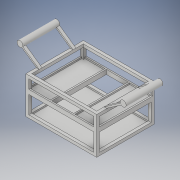
# Autodesk Inventor part: Battery Cart
Saved by Autodesk Inventor 2019.4 (Build 234330000, 330)
## iProperties
Created: 2019-09-11
Part Number: Battery Cart
Material: Generic
Document SubType Name: Modeling
Designer: josh
Density: 1 g/cm^3
Appearance: Default
Author: josh
Autodesk Inventor part; units mm, degrees
sketch "Sketch1" plane through (0, 0, 0) normal (1, 0, 0) x (0, 1, 0)
  line L0 (0, 0) -> (141.732, 0)
  line L1 (141.732, 0) -> (141.732, -495.3)
  line L2 (141.732, -495.3) -> (0, -495.3)
  line L3 (0, -495.3) -> (0, 0)
  dimension "d0" = 495.3
  dimension "d1" = 141.732
  constraints: 8 end point, 2 parallel, 1 horizontal, 1 perpendicular
  measures "d0" distance of L0.end L1.end
  measures "d1" distance of L1.end L2.end
extrude "Extrusion1" add sketch "Sketch1" along normal blind 609.6
shell "Shell1" thickness 25.4 removed faces 1 at (203.2, 141.732, -165.1)
sketch "Sketch2" plane through (0, 0, 0) normal (0, 0, 1) x (1, 0, 0)
  line L0 (25.4, 25.4) -> (25.4, 141.732) projected
  line L1 (584.2, 141.732) -> (584.2, 25.4) projected
  line L2 (25.4, 25.4) -> (584.2, 25.4)
  line L3 (584.2, 25.4) -> (584.2, 116.332)
  line L4 (584.2, 116.332) -> (25.4, 116.332)
  line L5 (25.4, 116.332) -> (25.4, 25.4)
  point P0 (0, 0)
  dimension "d5" = 90.932
  constraints: 8 end point, 2 parallel, 1 horizontal, 1 perpendicular, 1 point on line
  measures "d5" distance of L3.end L2.end
sketch "Sketch4" plane through (0, 0, 0) normal (-1, 0, 0) x (0, 0, 1)
  line L0 (-25.4, 141.732) -> (-25.4, 25.4) projected
  line L1 (-469.9, 25.4) -> (-469.9, 141.732) projected
  line L2 (-25.4, 25.4) -> (-469.9, 25.4)
  line L3 (-469.9, 25.4) -> (-469.9, 116.332)
  line L4 (-469.9, 116.332) -> (-25.4, 116.332)
  line L5 (-25.4, 116.332) -> (-25.4, 25.4)
  point P0 (0, 0)
  dimension "d13" = 90.932
  constraints: 8 end point, 2 parallel, 1 horizontal, 1 perpendicular, 1 point on line
  measures "d13" distance of L2.end L3.end
extrude "Extrusion6" cut sketch "Sketch4" against normal through all
extrude "Extrusion7" cut sketch "Sketch2" against normal through all
sketch "Sketch9" plane through (609.6, 25.4, -25.4) normal (0, 1, 0) x (1, 0, 0)
  line L0 (-609.6, -25.4) -> (-609.6, 469.9) projected
  line L1 (-609.6, 469.9) -> (0, 469.9) projected
  line L2 (0, 469.9) -> (0, -25.4) projected
  line L3 (-609.6, -25.4) -> (0, -25.4) projected
  line L4 (-609.6, 444.5) -> (-584.2, 444.5) projected
  line L5 (-596.9, 444.5) -> (-596.9, 0)
  line L6 (-609.6, 0) -> (-584.2, 0) projected
  line L7 (-584.2, 444.5) -> (-584.2, 469.9) projected
  line L8 (-584.2, 457.2) -> (-25.4, 457.2)
  line L9 (-25.4, 444.5) -> (-25.4, 469.9) projected
  line L10 (-25.4, 444.5) -> (0, 444.5) projected
  line L11 (-12.7, 444.5) -> (-12.7, 0)
  line L12 (-25.4, 0) -> (0, 0) projected
  line L13 (-584.2, -25.4) -> (-584.2, 0) projected
  line L14 (-584.2, -12.7) -> (-25.4, -12.7)
  line L15 (-25.4, -25.4) -> (-25.4, 0) projected
  line L16 (-609.6, 444.5) -> (-584.2, 444.5) projected
  line L17 (-596.9, 444.5) -> (-609.6, 444.5)
  line L18 (-609.6, 0) -> (-596.9, 0)
  line L19 (-609.6, 0) -> (-584.2, 0) projected
  line L20 (-25.4, 457.2) -> (-25.4, 469.9)
  line L21 (-609.6, 469.9) -> (0, 469.9) projected
  line L22 (-25.4, 444.5) -> (0, 444.5) projected
  line L23 (-12.7, 444.5) -> (0, 444.5)
  line L24 (-25.4, 457.2) -> (-25.4, 469.9)
  line L25 (-25.4, 0) -> (0, 0) projected
  line L26 (-12.7, 0) -> (0, 0)
  line L27 (-25.4, -12.7) -> (-25.4, -25.4)
  line L28 (-25.4, -25.4) -> (-584.2, -25.4) projected
  line L29 (-584.2, -25.4) -> (-584.2, -12.7)
  line L30 (-609.6, 444.5) -> (-609.6, 0)
  line L31 (-609.6, 469.9) -> (-609.6, -25.4) projected
  line L32 (-584.2, -25.4) -> (-25.4, -25.4)
  line L33 (-584.2, 469.9) -> (-25.4, 469.9) projected
  line L34 (-25.4, 469.9) -> (-584.2, 469.9)
  line L35 (0, 444.5) -> (0, 0) projected
  line L36 (0, 444.5) -> (0, 0)
  constraints: 32 end point, 8 midpoint, 6 collinear, 3 perpendicular, 2 horizontal, 1 parallel
extrude "Extrusion14" add sketch "Sketch9" along normal blind 12.7 contours L0 L4 L5 L6 | L13 L14 L15 L3 | L0 L1 L7 L4 | L1 L9 L8 L7 | L12 L11 L10 L2 | L1 L2 L10 L9
sketch "Sketch10" plane through (0, 0, -495.3) normal (0, -1, 0) x (1, 0, 0)
  line L0 (25.4, 469.9) -> (25.4, 25.4) projected
  line L1 (0, 495.3) -> (25.4, 495.3)
  line L2 (25.4, 495.3) -> (25.4, 469.9)
  line L3 (25.4, 469.9) -> (0, 469.9)
  line L4 (0, 469.9) -> (0, 495.3)
  line L5 (25.4, 25.4) -> (0, 25.4)
  line L6 (0, 25.4) -> (0, 0)
  line L7 (0, 0) -> (25.4, 0)
  line L8 (25.4, 0) -> (25.4, 25.4)
  line L9 (609.6, 0) -> (609.6, 495.3) projected
  line L10 (609.6, 0) -> (584.2, 0)
  line L11 (584.2, 0) -> (584.2, 25.4)
  line L12 (584.2, 25.4) -> (609.6, 25.4)
  line L13 (609.6, 25.4) -> (609.6, 0)
  line L14 (584.2, 469.9) -> (25.4, 469.9) projected
  line L15 (609.6, 495.3) -> (584.2, 495.3)
  line L16 (584.2, 495.3) -> (584.2, 469.9)
  line L17 (584.2, 469.9) -> (609.6, 469.9)
  line L18 (609.6, 469.9) -> (609.6, 495.3)
  dimension "d48" = 25.4
  dimension "d49" = 25.4
  dimension "d50" = 25.4
  dimension "d51" = 25.4
  dimension "d52" = 25.4
  dimension "d53" = 25.4
  dimension "d54" = 25.4
  dimension "d55" = 25.4
  constraints: 32 end point, 8 parallel, 4 horizontal, 4 perpendicular
  measures "d48" distance of L0.start L3.end
  measures "d49" distance of L1.end L0.start
  measures "d50" distance of L7.end L6.end
  measures "d51" distance of L6.end L5.end
  measures "d52" distance of L11.end L12.end
  measures "d53" distance of L10.end L11.end
  measures "d54" distance of L17.end L14.start
  measures "d55" distance of L14.start L15.end
extrude "Extrusion15" add sketch "Sketch10" along normal blind 152.4
sketch "Sketch11" plane through (0, -152.4, -495.3) normal (0, -1, 0) x (1, 0, 0)
  line L0 (609.6, 0) -> (609.6, 25.4) projected
  line L1 (0, 495.3) -> (609.6, 495.3)
  line L2 (609.6, 495.3) -> (609.6, 0)
  line L3 (609.6, 0) -> (0, 0)
  line L4 (0, 0) -> (0, 495.3)
  constraints: 8 end point, 2 parallel, 1 horizontal, 1 perpendicular
extrude "Extrusion16" add sketch "Sketch11" along normal blind 25.4
sketch "Sketch12" plane through (25.4, 25.4, -12.7) normal (0, 1, 0) x (1, 0, 0)
  line L0 (185.42, 457.2) -> (185.42, 12.7)
  line L1 (373.38, 457.2) -> (373.38, 12.7)
  line L2 (373.38, 457.2) -> (373.38, 12.7)
  line L3 (185.42, 12.7) -> (185.42, 457.2)
  line L4 (373.38, 457.2) -> (373.38, 469.9)
  line L5 (185.42, 469.9) -> (185.42, 457.2)
  line L6 (185.42, 12.7) -> (185.42, 1.0295)
  line L7 (373.38, 1.0295) -> (373.38, 12.7)
  line L8 (185.42, 469.9) -> (373.38, 469.9)
  line L9 (373.38, 469.9) -> (373.38, 1.0295)
  line L10 (373.38, 1.0295) -> (185.42, 1.0295)
  line L11 (185.42, 1.0295) -> (185.42, 469.9)
  line L12 (558.8, 0) -> (0, 0) projected
  line L13 (185.42, 469.9) -> (172.72, 469.9)
  line L14 (172.72, 469.9) -> (172.72, 0)
  line L15 (172.72, 0) -> (185.42, 0)
  line L16 (185.42, 0) -> (185.42, 469.9)
  line L17 (373.38, 469.9) -> (386.08, 469.9)
  line L18 (386.08, 469.9) -> (386.08, -5.7755)
  line L19 (386.08, -5.7755) -> (373.38, -5.7755)
  line L20 (373.38, -5.7755) -> (373.38, 469.9)
  dimension "d64" = 12.7
  dimension "d65" = 12.7
  constraints: 40 end point, 9 parallel, 3 horizontal, 3 perpendicular, 2 point on line
  measures "d64" distance of L15.end L14.end
  measures "d65" distance of L18.end L19.end
extrude "Extrusion17" cut sketch "Sketch12" against normal blind 25.4 contours L5 L8 L4 L1 L7 L10 L6 L0
extrude "Extrusion18" add sketch "Sketch12" along normal blind 12.7 contours L0 L6 L16 L12 L14 L13 L5 | L17 L18 L12 L20 L7 L1 L4 | L12 L18 L19 L20
sketch "Sketch13" plane through (0, -152.4, -495.3) normal (0, 1, 0) x (1, 0, 0)
  line L0 (609.6, -495.3) -> (0, -495.3) projected
  line L1 (609.6, 0) -> (609.6, -495.3) projected
  line L2 (0, -495.3) -> (0, 0) projected
  line L3 (0, 0) -> (609.6, 0) projected
  line L4 (584.2, -25.4) -> (584.2, -469.9)
  line L5 (584.2, -469.9) -> (25.4, -469.9)
  line L6 (25.4, -469.9) -> (25.4, -25.4)
  line L7 (25.4, -25.4) -> (584.2, -25.4)
  dimension "d68" = 25.4
  constraints: 8 end point, 3 other
  measures "d68" distance between parallel lines of L3 L7
extrude "Extrusion19" cut sketch "Sketch13" against normal blind 12.7 contours L4 L5 L6 L7
ref_plane "Work Plane1" through (609.6, 141.732, -393.7) normal (0, 0, -1) x (-1, 0, 0)
ref_plane "Work Plane2" through (0, 141.732, -101.6) normal (0, 0, 1) x (1, 0, 0)
sketch "Sketch14" plane through (0, 141.732, -101.6) normal (0, 0, 1) x (1, 0, 0)
  line L0 (584.2, 0) -> (25.4, 0) projected
  line L1 (16.946, -12.0735) -> (25.4, 0)
  line L2 (25.4, 0) -> (228.6, 0) construction
  line L3 (25.4, 0) -> (-141.0517, 116.5507)
  line L4 (-141.0517, 116.5507) -> (-148.3361, 106.1475)
  line L5 (-148.3361, 106.1475) -> (18.1156, -10.4032)
  line L6 (18.1156, -10.4032) -> (25.4, 0)
  line L7 (25.4, 0) -> (228.6, 0) construction
  point P0 (0, -141.732)
  dimension "d75" = 203.2
  dimension "d76" = 145
  dimension "d77" = 12.7
  constraints: 14 end point, 2 horizontal, 2 parallel, 1 equal length, 1 perpendicular
  measures "d75" distance of L0.end L3.end
  measures "d76" angle of L7 L3
  measures "d77" distance of L4.end L3.end
sketch "Sketch15" plane through (609.6, 141.732, -393.7) normal (0, 0, -1) x (-1, 0, 0)
  line L0 (584.2, 0) -> (750.6517, 116.5507) projected
  line L1 (757.9361, 106.1475) -> (591.4844, -10.4032) projected
  line L2 (750.6517, 116.5507) -> (757.9361, 106.1475) projected
  line L3 (584.2, 0) -> (750.6517, 116.5507)
  line L4 (750.6517, 116.5507) -> (757.9361, 106.1475)
  line L5 (757.9361, 106.1475) -> (591.4844, -10.4032)
  line L6 (591.4844, -10.4032) -> (584.2, 0)
  point P0 (609.6, -141.732)
  constraints: 8 end point, 2 parallel, 1 perpendicular
extrude "Extrusion20" add sketch "Sketch15" along normal mid plane 25.4
extrude "Extrusion21" add sketch "Sketch14" along normal mid plane 25.4
ref_plane "Work Plane3" through (304.8, 0, 0) normal (1, 0, 0) x (0, 0, -1)
sketch "Sketch16" plane through (609.6, 141.732, -406.4) normal (0, 0, -1) x (-1, 0, 0)
  circle A0 centre (749.0923, 107.7069) radius 25.4
  point P0 (609.6, -141.732)
  point P1 (750.6517, 116.5507)
  point P2 (757.9361, 106.1475)
  constraints: 1 centre point
extrude "Extrusion24" add sketch "Sketch16" against normal up to surface (317.5 mm away)
mirror "Mirror2" about plane through (304.8, 0, 0) normal (1, 0, 0) of "Extrusion24", "Extrusion21", "Extrusion20"
sketch "Sketch17" plane through (584.2, 116.332, -469.9) normal (0, 0, 1) x (1, 0, 0)
  line L0 (12.7, -78.232) -> (25.4, -78.232) projected
  line L1 (25.4, 0) -> (25.4, -78.232) projected
  line L2 (0, 0) -> (25.4, 0) projected
  line L3 (0, 0) -> (0, -90.932) projected
  line L4 (0, -90.932) -> (12.7, -90.932) projected
  line L5 (12.7, -90.932) -> (12.7, -78.232) projected
  point P0 (-584.2, -116.332)
extrude "Extrusion25" cut sketch "Sketch17" against normal blind 12.7
sketch "Sketch18" plane through (584.2, 38.1, -482.6) normal (-1, 0, 0) x (0, 0, 1)
  line L0 (0, 0) -> (0, 78.232) projected
  line L1 (0, 78.232) -> (-12.7, 78.232) projected
  line L2 (-12.7, 0) -> (-12.7, 78.232) projected
  line L3 (-12.7, 0) -> (0, 0) projected
  point P0 (482.6, -38.1)
extrude "Extrusion26" cut sketch "Sketch18" against normal blind 12.7
body "Solid1"
